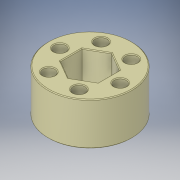
# Autodesk Inventor part: am-1305
Saved by Autodesk Inventor 2017.1 (Build 211199000, 199)
## iProperties
Category: Spacer
Company: Autodesk Inc.
Created: 2016-12-22
Part Number: am-1305
Material: Polypropylene
Document SubType Name: Modeling
Designer: Autodesk Inc.
Density: 0.899 g/cm^3
Appearance: Smooth - Ash
Catalog Web Link: http://www.andymark.com/product-p/am-1305.htm
Vendor: Andy Mark Inc.
Author: Autodesk Inc.
Keywords: Drive Base Kit
Autodesk Inventor part; units mm, degrees
ref_plane "YZ Plane" through (0, 0, 0) normal (1, 0, 0) x (0, 1, 0)
ref_plane "XZ Plane" through (0, 0, 0) normal (0, 1, 0) x (-1, 0, 0)
ref_plane "XY Plane" through (0, 0, 0) normal (0, 0, 1) x (1, 0, 0)
sketch "Sketch1" plane through (0, 0, 0) normal (0, 1, 0) x (-1, 0, 0)
  circle A0 centre (0, 0) radius 14.2748
  dimension "d0" = 28.5496
  constraints: 1 centre point, 1 coincident
  measures "d0" diameter of A0
extrude "Extrusion1" add sketch "Sketch1" against normal blind 14.478
sketch "Sketch2" plane through (0, 0, 0) normal (0, 1, 0) x (1, 0, 0)
  circle A0 centre (0, 0) radius 10.287
  circle A1 centre (-10.287, 0) radius 2.032
  dimension "d3" = 20.574
  dimension "d4" = 4.064
  constraints: 1 centre point, 1 coincident, 1 horizontal alignment, 2 other
  measures "d4" diameter of A1
extrude "Extrusion2" cut sketch "Sketch2" against normal up to next contours A1 A0 | A0 A1 picked at (-9.5948, 0) picked at (-10.9494, 0)
chamfer "Chamfer1" distance 0.254 angle 45 2 edges at (-12.319, 0, 0) (-12.319, -14.478, 0)
pattern_circular "Circular Pattern1" count 6 over 360 about axis through (0, 0, 0) along (0, -1, 0) of "Extrusion2", "Chamfer1"
chamfer "Chamfer2" distance 0.254 angle 45 2 edges at (14.2748, 0, 0) (14.2748, -14.478, 0)
sketch "Sketch3" plane through (0, 0, 0) normal (0, 1, 0) x (1, 0, 0)
  line L0 (-6.3754, 3.6808) -> (0, 7.3617)
  line L1 (0, 7.3617) -> (6.3754, 3.6808)
  line L2 (6.3754, 3.6808) -> (6.3754, -3.6808)
  line L3 (6.3754, -3.6808) -> (0, -7.3617)
  line L4 (0, -7.3617) -> (-6.3754, -3.6808)
  line L5 (-6.3754, -3.6808) -> (-6.3754, 3.6808)
  point P0 (0, 0)
  point P1 (0, 0)
  dimension "d16" = 12.7508
  constraints: 12 end point, 1 coincident, 1 vertical, 13 other
  measures "d16" distance of L1.end L0.start
extrude "Extrusion3" cut sketch "Sketch3" against normal up to next
chamfer "Chamfer3" distance 0.254 angle 45 12 edges at (-6.3754, 0, 0) (-3.1877, 0, -5.5213) (3.1877, 0, -5.5213) (6.3754, 0, 0) (3.1877, 0, 5.5213) (-3.1877, 0, 5.5213) (3.1877, -14.478, 5.5213) (6.3754, -14.478, 0) (3.1877, -14.478, -5.5213) (-3.1877, -14.478, -5.5213) (-6.3754, -14.478, 0) (-3.1877, -14.478, 5.5213)
body "Solid1"
